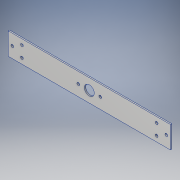
# Autodesk Inventor part: slider-crossbeam
Saved by Autodesk Inventor 2017 (Build 210142000, 142)
## iProperties
Created: 2017-12-27
Part Number: slider-crossbeam
Material: Aluminum 6061
Document SubType Name: Modeling
Designer: Micah
Density: 2.7 g/cm^3
Appearance: Aluminum - Flat
Mass: 169.821 g
Surface Area: 428.225 cm^2
Volume: 62.8966 cm^3
Author: Micah
Autodesk Inventor part; units mm, degrees
ref_plane "YZ Plane" through (0, 0, 0) normal (1, 0, 0) x (0, 1, 0)
ref_plane "XZ Plane" through (0, 0, 0) normal (0, 1, 0) x (-1, 0, 0)
ref_plane "XY Plane" through (0, 0, 0) normal (0, 0, 1) x (1, 0, 0)
sketch "Sketch1" plane through (0, 0, 0) normal (0, 0, 1) x (1, 0, 0)
  line L0 (355.6, 50.8) -> (-19.05, 50.8)
  line L1 (12.7, 50.8) -> (12.7, 0) construction
  line L2 (0, 38.1) -> (12.7, 38.1) construction
  line L3 (0, 12.7) -> (12.7, 12.7) construction
  circle A0 centre (12.7, 38.1) radius 3.175
  circle A1 centre (12.7, 12.7) radius 3.175
  line L4 (168.275, 50.8) -> (168.275, 0) construction
  line L5 (-19.05, 50.8) -> (-19.05, 0)
  line L6 (355.6, 50.8) -> (355.6, 0)
  circle A2 centre (-9.525, 25.4) radius 3.175
  circle A3 centre (323.85, 38.1) radius 3.175
  circle A4 centre (323.85, 12.7) radius 3.175
  line L7 (355.6, 50.8) -> (355.6, 0)
  circle A5 centre (346.075, 25.4) radius 3.175
  line L8 (-19.05, 0) -> (355.6, 0)
  dimension "d0" = 374.65
  dimension "d3" = 12.7
  dimension "d4" = 25.4
  dimension "d5" = 6.35
  dimension "d6" = 6.35
  dimension "d10" = 6.35
  dimension "d11" = 31.75
  constraints: 18 end point, 6 centre point, 5 point on line, 5 symmetric about line, 2 coincident, 2 perpendicular, 1 horizontal, 1 midpoint, 3 other
  measures "d0" distance of L0.end L0.start
  measures "d3" distance between parallel lines of L0 L2
  measures "d4" distance between parallel lines of L3 L2
  measures "d5" diameter of A0
  measures "d6" diameter of A1
  measures "d10" diameter of A2
  measures "d11" distance between parallel lines of L5 L1
extrude "Extrusion2" add sketch "Sketch1" along normal blind 3.175
sketch "Sketch3" plane through (0, 0, 3.175) normal (0, 0, 1) x (1, 0, 0)
  line L0 (-19.05, 50.8) -> (-19.05, 0) projected
  line L1 (-19.05, 25.4) -> (168.275, 25.4)
  line L2 (355.6, 50.8) -> (-19.05, 50.8) projected
  line L3 (168.275, 25.4) -> (168.275, 50.8)
  point P0 (0, 0)
  constraints: 4 end point, 2 midpoint, 1 parallel
hole "Hole1" at (168.275, 25.4, 3.175) direction (0, 0, -1) diameter 22.86 depth 25.4 tip angle 118
sketch "Sketch4" plane through (0, 0, 3.175) normal (0, 0, 1) x (1, 0, 0)
  circle A0 centre (168.275, 25.4) radius 11.43 projected
  line L0 (168.275, 25.4) -> (142.875, 25.4)
  circle A1 centre (142.875, 25.4) radius 3.175
  line L1 (355.6, 50.8) -> (-19.05, 50.8) projected
  line L2 (168.275, 50.8) -> (168.275, 0)
  circle A2 centre (193.675, 25.4) radius 3.175
  point P0 (0, 0)
  dimension "d21" = 25.4
  dimension "d22" = 6.35
  constraints: 4 end point, 2 centre point, 1 coincident, 1 horizontal, 1 midpoint, 1 symmetric about line, 1 vertical, 1 other
  measures "d21" distance of L0.start L0.end
  measures "d22" diameter of A1
hole "Hole2" at (193.675, 25.4, 3.175) at (142.875, 25.4, 3.175) direction (0, 0, -1) diameter 6.35 depth 25.4 tip angle 118
body "Solid2"
